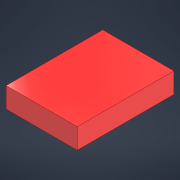
# Autodesk Inventor part: Boost-Buck-Converter
Saved by Autodesk Inventor 2022 (Build 260153000, 153)
## iProperties
Created: 2024-05-10
Part Number: Boost-Buck-Converter
Material: Generic
Document SubType Name: Modeling
Designer: jo_ki
Density: 1 g/cm^3
Appearance: Light Red
Author: jo_ki
Autodesk Inventor part; units mm, degrees
ref_plane "YZ Plane" through (0, 0, 0) normal (1, 0, 0) x (0, 1, 0)
ref_plane "XZ Plane" through (0, 0, 0) normal (0, 1, 0) x (-1, 0, 0)
ref_plane "XY Plane" through (0, 0, 0) normal (0, 0, 1) x (1, 0, 0)
sketch "Sketch1" plane through (0, 0, 0) normal (0, 1, 0) x (-1, 0, 0)
  line L0 (-7, 9.5) -> (7, 9.5)
  line L1 (7, 9.5) -> (7, -9.5)
  line L2 (7, -9.5) -> (-7, -9.5)
  line L3 (-7, -9.5) -> (-7, 9.5)
  line L4 (-7, 9.5) -> (7, -9.5) construction
  line L5 (7, 9.5) -> (-7, -9.5) construction
  point P0 (0, 0)
  dimension "d0" = 19
  dimension "d1" = 14
  constraints: 12 end point, 2 midpoint, 2 parallel, 1 horizontal, 1 perpendicular
  measures "d0" distance of L0.end L1.end
  measures "d1" distance of L1.end L2.end
extrude "Extrusion1" add sketch "Sketch1" along normal blind 4
body "Solid1"
